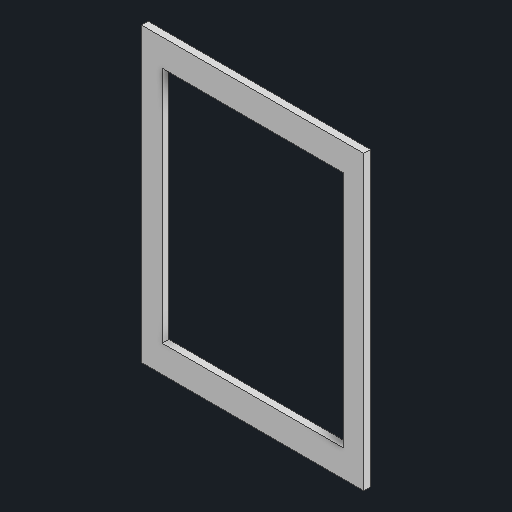
# Autodesk Inventor part: Pieza11
Saved by Autodesk Inventor 2026.1 (Build 301233020, 233B)
## iProperties
Created: 2026-05-06
Part Number: Pieza11
Material: Genérico
Document SubType Name: Modeling
Designer: OlmesTech
Density: 1 g/cm^3
Appearance: Valor por defecto
Author: OlmesTech
Autodesk Inventor part; units mm, degrees
ref_plane "YZ Plane" through (0, 0, 0) normal (1, 0, 0) x (0, 1, 0)
ref_plane "XZ Plane" through (0, 0, 0) normal (0, 1, 0) x (-1, 0, 0)
ref_plane "XY Plane" through (0, 0, 0) normal (0, 0, 1) x (1, 0, 0)
sketch "Boceto1" plane through (0, 0, 0) normal (0, 0, 1) x (1, 0, 0)
  line L0 (-2.971, -130) -> (-104.8493, -130) projected
  line L1 (-2.6867, 0) -> (-104.8493, 0) projected
  line L2 (0, 0) -> (0, -127) projected
  line L3 (0, -130) -> (0, -127) projected
  line L4 (5.5477, -130) -> (-2.971, -130) projected
  line L5 (5.5477, 0) -> (-2.6867, 0) projected
  line L6 (-98.8843, -130) -> (-98.8843, 0)
  line L7 (-98.8843, -130) -> (0, 0)
  line L8 (-98.8843, 0) -> (0, -130)
  line L9 (-9.1278, -118) -> (-89.7565, -118)
  line L10 (-89.7565, -118) -> (-89.7565, -12)
  line L11 (-89.7565, -12) -> (-9.1278, -12)
  line L12 (-9.1278, -12) -> (-9.1278, -118)
  line L13 (-9.1278, -118) -> (-89.7565, -12) construction
  line L14 (-89.7565, -118) -> (-9.1278, -12) construction
  point P0 (-49.4421, -65)
  dimension "d2" = 12
  constraints: 18 end point, 3 midpoint, 3 point on line, 2 parallel, 2 perpendicular, 1 horizontal
  measures "d2" distance between parallel lines of L1 L11
extrude "Extrusión1" add sketch "Boceto1" along normal blind 3 contours L0 L7 L9 L8 L4 | L6 L8 L10 L7 | L8 L12 L7 L2 L3 | L1 L5 L7 L11 L8
